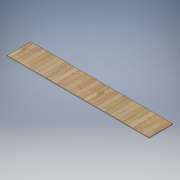
# Autodesk Inventor part: Wand
Saved by Autodesk Inventor 2019 (Build 230136000, 136)
## iProperties
Created: 2021-09-27
Part Number: Wand
Material: Holz (Ahorn)
Document SubType Name: Modeling
Designer: mritt
Density: 0.67 g/cm^3
Appearance: Ahorn - natur - glänzend - dunkel getönt
Author: mritt
Autodesk Inventor part; units mm, degrees
ref_plane "YZ Plane" through (0, 0, 0) normal (1, 0, 0) x (0, 1, 0)
ref_plane "XZ Plane" through (0, 0, 0) normal (0, 1, 0) x (-1, 0, 0)
ref_plane "XY Plane" through (0, 0, 0) normal (0, 0, 1) x (1, 0, 0)
sketch "Skizze1" plane through (0, 0, 0) normal (0, 1, 0) x (-1, 0, 0)
  line L0 (2221.4286, -2042.8572) -> (421.4286, -2042.8572)
  line L1 (421.4286, -2042.8572) -> (421.4286, -2342.8572)
  line L2 (421.4286, -2342.8572) -> (2221.4286, -2342.8572)
  line L3 (2221.4286, -2342.8572) -> (2221.4286, -2042.8572)
  point P0 (0, 0)
  dimension "d0" = 1800
  dimension "d1" = 300
  constraints: 8 end point, 2 parallel, 1 horizontal, 1 perpendicular
  measures "d0" distance of L1.end L2.end
  measures "d1" distance of L2.end L0.start
extrude "Extrusion1" add sketch "Skizze1" along normal blind 10
